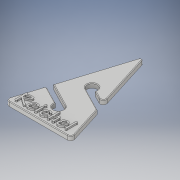
# Autodesk Inventor part: arrow_copied
Saved by Autodesk Inventor 2019 (Build 230136000, 136)
## iProperties
Created: 2019-04-04
Part Number: arrow_copied
Material: Generic
Document SubType Name: Modeling
Designer: jmc
Density: 1 g/cm^3
Appearance: Default
Author: jmc
Autodesk Inventor part; units mm, degrees
ref_plane "YZ Plane" through (0, 0, 0) normal (1, 0, 0) x (0, 1, 0)
ref_plane "XZ Plane" through (0, 0, 0) normal (0, 1, 0) x (-1, 0, 0)
ref_plane "XY Plane" through (0, 0, 0) normal (0, 0, 1) x (1, 0, 0)
sketch "Sketch1" plane through (0, 0, 0) normal (0, 1, 0) x (-1, 0, 0)
  line L0 (18.6404, 33.842) -> (-18.6393, 33.842)
  arc A0 (-0.9051, -31.4569) -> (1.0039, -31.4556) centre (0.0492, -31.158) ccw
  line L1 (-11.041, 0.8979) -> (-0.9051, -31.4569)
  line L2 (14.0042, 10.2488) -> (1.0039, -31.4556)
  arc A1 (20.5497, 31.2468) -> (18.6404, 33.842) centre (18.6404, 31.842) ccw
  arc A2 (-18.6393, 33.842) -> (-20.5478, 31.2441) centre (-18.6393, 31.842) ccw
  arc A3 (3.0063, 19.9469) -> (-1.4629, 18.1957) centre (-0.0005, 21.042) ccw
  arc A4 (-3.0072, 0.5972) -> (1.4619, 2.3483) centre (-0.0005, -0.498) ccw
  line L3 (14.0339, 14.281) -> (3.0063, 19.9469)
  line L4 (-1.4629, 18.1957) -> (14.0042, 10.2488)
  line L5 (20.5497, 31.2468) -> (15.4456, 14.8728)
  line L6 (14.0042, 10.2488) -> (1.0039, -31.4556)
  line L7 (1.4619, 2.3483) -> (-13.9812, 10.2829)
  line L8 (-3.0072, 0.5972) -> (-8.2185, 3.2747)
  line L9 (-20.5478, 31.2441) -> (-13.9812, 10.2829)
  line L10 (-11.041, 0.8979) -> (-0.9051, -31.4569)
  arc A5 (14.0339, 14.281) -> (15.4456, 14.8728) centre (14.4909, 15.1704) ccw
  arc A6 (-8.2185, 3.2747) -> (-11.041, 0.8979) centre (-9.1325, 1.4958) ccw
  point P0 (-0.0005, -4.3624)
  point P1 (-0.0005, -4.3624)
  point P2 (20.9995, 33.842)
  point P3 (21.3587, 33.842)
  point P4 (-21.3617, 33.842)
  point P5 (-0.0005, -4.3624)
  point P6 (-0.0005, 33.842)
  point P7 (-0.0005, -4.3624)
  point P8 (15.0916, 13.7375)
  point P9 (-12.47, 5.4591)
  dimension "d3" = 1
  dimension "d26" = 2
  dimension "d27" = 6.4
  dimension "d28" = 12.8
  dimension "d30" = 6.4
  dimension "d31" = 21.54
  dimension "d33" = 3.6
  dimension "d35" = 3.6
  dimension "d38" = 1
  dimension "d39" = 2
  constraints: 22 end point, 18 tangent, 14 point on circle, 9 point on line, 7 centre point, 3 coincident, 3 parallel, 1 equal radius, 1 horizontal
  measures "d3" radius of A0
  measures "d26" radius of A1
  measures "d27" diameter of A3
  measures "d28" distance from line of A3.centre L0
  measures "d30" diameter of A4
  measures "d31" distance of A4.centre A3.centre
  measures "d33" distance between parallel lines of L3 L4
  measures "d35" distance between parallel lines of L7 L8
  measures "d38" radius of A5
  measures "d39" radius of A6
extrude "Extrusion1" add sketch "Sketch1" along normal blind 2.8
sketch "Sketch2" plane through (0, 2.8, 0) normal (0, 1, 0) x (1, 0, 0)
  line L0 (-17.863, -24.2841) -> (16.586, -24.2841) construction
  line L1 (16.586, -24.2841) -> (16.586, -32.2942) construction
  line L2 (16.586, -32.2942) -> (-17.863, -32.2942) construction
  line L3 (-17.863, -32.2942) -> (-17.863, -24.2841) construction
  spline S0 degree 2 poles (-17.1698, -31.489) (-17.1698, -31.7411) (-16.9037, -32.1122) (-16.6096, -32.1192) knots 0 0 0 1 2 2 2
  spline S1 degree 2 poles (-16.6096, -32.1192) (-16.2946, -32.1262) (-15.8114, -31.8671) (-15.7974, -31.524) knots 0 0 0 1 2 2 2
  spline S2 degree 2 poles (-15.7974, -31.524) (-15.7974, -31.419) (-15.8744, -31.2159) (-15.9025, -31.1599) knots 0 0 0 1 2 2 2
  line L4 (-15.9025, -31.1599) -> (-15.9025, -28.8563)
  line L5 (-15.9025, -28.8563) -> (-11.7504, -31.8811)
  spline S3 degree 2 poles (-11.7504, -31.8811) (-11.6664, -32.0421) (-11.3653, -32.2032) (-11.1902, -32.2032) knots 0 0 0 1 2 2 2
  spline S4 degree 2 poles (-11.1902, -32.2032) (-10.9242, -32.2032) (-10.497, -31.8531) (-10.483, -31.51) knots 0 0 0 1 2 2 2
  spline S5 degree 2 poles (-10.483, -31.51) (-10.497, -31.2789) (-10.9452, -30.9359) (-11.2532, -31.0339) knots 0 0 0 1 2 2 2
  line L6 (-11.2532, -31.0339) -> (-15.0832, -28.2682)
  spline S6 degree 2 poles (-15.0832, -28.2682) (-13.2768, -27.9461) (-11.3653, -26.5947) (-11.3583, -25.6845) knots 0 0 0 1 2 2 2
  spline S7 degree 2 poles (-11.3583, -25.6845) (-11.3723, -25.0963) (-12.2685, -24.4662) (-13.0037, -24.4592) knots 0 0 0 1 2 2 2
  spline S8 degree 2 poles (-13.0037, -24.4592) (-13.7109, -24.4592) (-15.1533, -24.7813) (-15.9025, -25.1173) knots 0 0 0 1 2 2 2
  line L7 (-15.9025, -25.1173) -> (-15.9025, -24.9983)
  spline S9 degree 2 poles (-15.9025, -24.9983) (-15.8184, -24.6972) (-16.1405, -24.3261) (-16.4206, -24.3191) knots 0 0 0 1 2 2 2
  spline S10 degree 2 poles (-16.4206, -24.3191) (-16.6937, -24.3191) (-17.0858, -24.6132) (-17.0998, -24.8723) knots 0 0 0 1 2 2 2
  spline S11 degree 2 poles (-17.0998, -24.8723) (-17.0928, -24.9633) (-17.0437, -25.1524) (-17.0157, -25.2154) knots 0 0 0 1 2 2 2
  line L8 (-17.0157, -25.2154) -> (-17.0157, -25.4674)
  spline S12 degree 2 poles (-17.0157, -25.4674) (-17.1698, -25.5165) (-17.3798, -25.8315) (-17.3798, -26.1256) knots 0 0 0 1 2 2 2
  spline S13 degree 2 poles (-17.3798, -26.1256) (-17.3728, -26.3567) (-17.2118, -26.5807) (-17.1208, -26.5737) knots 0 0 0 1 2 2 2
  spline S14 degree 2 poles (-17.1208, -26.5737) (-17.0858, -26.5807) (-17.0367, -26.5667) (-17.0157, -26.5527) knots 0 0 0 1 2 2 2
  line L9 (-17.0157, -26.5527) -> (-17.0157, -31.1109)
  spline S15 degree 2 poles (-17.0157, -31.1109) (-17.0648, -31.1879) (-17.1628, -31.398) (-17.1698, -31.489) knots 0 0 0 1 2 2 2
  spline S16 degree 2 poles (-15.9025, -26.0276) (-15.1463, -25.6775) (-13.8159, -25.3834) (-13.3118, -25.3904) knots 0 0 0 1 2 2 2
  spline S17 degree 2 poles (-13.3118, -25.3904) (-12.9547, -25.3904) (-12.5416, -25.6355) (-12.5416, -25.8525) knots 0 0 0 1 2 2 2
  spline S18 degree 2 poles (-12.5416, -25.8525) (-12.5486, -26.2796) (-13.4518, -26.9588) (-14.9712, -27.491) (-15.9025, -27.687) knots 0 0 0 1 2 3 3 3
  line L10 (-15.9025, -27.687) -> (-15.9025, -26.0276)
  spline S19 degree 2 poles (-7.2132, -26.8118) (-8.0044, -26.8188) (-9.4048, -27.792) (-10.294, -29.4865) (-10.308, -30.5998) knots 0 0 0 1 2 3 3 3
  spline S20 degree 2 poles (-10.308, -30.5998) (-10.294, -31.496) (-9.3067, -32.2592) (-8.5365, -32.2522) knots 0 0 0 1 2 2 2
  spline S21 degree 2 poles (-8.5365, -32.2522) (-7.8084, -32.2382) (-6.7021, -31.8181) (-5.9529, -31.2159) (-5.5748, -30.6698) (-5.5748, -30.5368) knots 0 0 0 1 2 3 4 4 4
  spline S22 degree 2 poles (-5.5748, -30.5368) (-5.5678, -30.3477) (-5.7848, -30.0256) (-6.1069, -30.0186) knots 0 0 0 1 2 2 2
  spline S23 degree 2 poles (-6.1069, -30.0186) (-6.401, -30.0256) (-6.7161, -30.3267) (-6.6951, -30.5368) knots 0 0 0 1 2 2 2
  spline S24 degree 2 poles (-6.6951, -30.5368) (-6.8071, -30.7048) (-7.2972, -31.0689) (-7.9974, -31.321) (-8.4105, -31.328) knots 0 0 0 1 2 3 3 3
  spline S25 degree 2 poles (-8.4105, -31.328) (-8.7956, -31.335) (-9.2227, -30.9429) (-9.2227, -30.5017) knots 0 0 0 1 2 2 2
  spline S26 degree 2 poles (-9.2227, -30.5017) (-9.2227, -30.3267) (-9.1877, -30.0046) (-9.1387, -29.8646) knots 0 0 0 1 2 2 2
  line L11 (-9.1387, -29.8646) -> (-8.5996, -29.7666)
  spline S27 degree 2 poles (-8.5996, -29.7666) (-7.5773, -29.5915) (-6.331, -29.2204) (-5.7008, -28.8493) (-5.4837, -28.4712) (-5.4908, -28.2682) knots 0 0 0 1 2 3 4 4 4
  spline S28 degree 2 poles (-5.4908, -28.2682) (-5.4837, -28.0231) (-5.7988, -27.3509) (-6.555, -26.8258) (-7.2132, -26.8118) knots 0 0 0 1 2 3 3 3
  spline S29 degree 2 poles (-7.2622, -27.715) (-6.8771, -27.729) (-6.534, -28.0931) (-6.541, -28.3172) knots 0 0 0 1 2 2 2
  spline S30 degree 2 poles (-6.541, -28.3172) (-6.527, -28.4012) (-6.8631, -28.5902) (-7.8924, -28.8423) (-8.9286, -29.0244) knots 0 0 0 1 2 3 3 3
  spline S31 degree 2 poles (-8.9286, -29.0244) (-8.6556, -28.4502) (-7.7733, -27.729) (-7.2622, -27.715) knots 0 0 0 1 2 2 2
  spline S32 degree 2 poles (-3.1942, -27.4349) (-3.2012, -27.2389) (-3.5583, -26.8958) (-3.7753, -26.8818) knots 0 0 0 1 2 2 2
  spline S33 degree 2 poles (-3.7753, -26.8818) (-4.1254, -26.8888) (-4.4475, -27.0849) (-4.5245, -27.3999) (-4.5175, -27.568) knots 0 0 0 1 2 3 3 3
  spline S34 degree 2 poles (-4.5175, -27.568) (-4.5175, -27.652) (-4.4685, -27.82) (-4.4125, -27.8761) knots 0 0 0 1 2 2 2
  line L12 (-4.4125, -27.8761) -> (-4.4125, -31.1599)
  spline S35 degree 2 poles (-4.4125, -31.1599) (-4.4545, -31.2019) (-4.5525, -31.405) (-4.5525, -31.566) knots 0 0 0 1 2 2 2
  spline S36 degree 2 poles (-4.5525, -31.566) (-4.5525, -31.8251) (-4.2584, -32.1192) (-4.0204, -32.1192) knots 0 0 0 1 2 2 2
  spline S37 degree 2 poles (-4.0204, -32.1192) (-3.8313, -32.1192) (-3.4392, -31.9931) (-3.1661, -31.7411) (-3.1591, -31.538) knots 0 0 0 1 2 3 3 3
  spline S38 degree 2 poles (-3.1591, -31.538) (-3.1661, -31.433) (-3.2642, -31.2439) (-3.3132, -31.2089) knots 0 0 0 1 2 2 2
  line L13 (-3.3132, -31.2089) -> (-3.3132, -27.827)
  spline S39 degree 2 poles (-3.3132, -27.827) (-3.2922, -27.778) (-3.2012, -27.589) (-3.1942, -27.4349) knots 0 0 0 1 2 2 2
  spline S40 degree 2 poles (-3.7053, -24.6272) (-4.0414, -24.6412) (-4.4125, -25.2434) (-4.4125, -25.7055) knots 0 0 0 1 2 2 2
  spline S41 degree 2 poles (-4.4125, -25.7055) (-4.4125, -25.9576) (-4.1604, -26.2656) (-3.8803, -26.2726) knots 0 0 0 1 2 2 2
  spline S42 degree 2 poles (-3.8803, -26.2726) (-3.5933, -26.2656) (-3.1802, -25.6985) (-3.1732, -25.1734) knots 0 0 0 1 2 2 2
  spline S43 degree 2 poles (-3.1732, -25.1734) (-3.1732, -24.9143) (-3.4462, -24.6272) (-3.7053, -24.6272) knots 0 0 0 1 2 2 2
  spline S44 degree 2 poles (0.7829, -26.8118) (0.4608, -26.8188) (-0.2324, -27.0779) (-0.8275, -27.463) (-0.9956, -27.659) knots 0 0 0 1 2 3 3 3
  spline S45 degree 2 poles (-0.9956, -27.659) (-1.3527, -28.0091) (-1.8988, -28.7513) (-2.2069, -29.7035) (-2.2139, -30.3757) knots 0 0 0 1 2 3 3 3
  spline S46 degree 2 poles (-2.2139, -30.3757) (-2.2069, -31.2229) (-1.1986, -32.2732) (-0.3164, -32.2872) knots 0 0 0 1 2 2 2
  spline S47 degree 2 poles (-0.3164, -32.2872) (0.2297, -32.2872) (1.098, -31.9861) (1.4691, -31.6851) knots 0 0 0 1 2 2 2
  spline S48 degree 2 poles (1.4691, -31.6851) (1.8121, -31.433) (2.2673, -30.8588) (2.4983, -30.3967) (2.4983, -30.3267) knots 0 0 0 1 2 3 3 3
  spline S49 degree 2 poles (2.4983, -30.3267) (2.5053, -30.1797) (2.2533, -29.8436) (1.9242, -29.8296) knots 0 0 0 1 2 2 2
  spline S50 degree 2 poles (1.9242, -29.8296) (1.6441, -29.8366) (1.441, -30.1447) (1.399, -30.3827) knots 0 0 0 1 2 2 2
  spline S51 degree 2 poles (1.399, -30.3827) (1.28, -30.6068) (0.9019, -30.9779) (0.7059, -31.0969) knots 0 0 0 1 2 2 2
  spline S52 degree 2 poles (0.7059, -31.0969) (0.5238, -31.2019) (0.1527, -31.342) (-0.0503, -31.342) knots 0 0 0 1 2 2 2
  spline S53 degree 2 poles (-0.0503, -31.342) (-0.5895, -31.335) (-1.1286, -30.7398) (-1.1286, -30.1937) knots 0 0 0 1 2 2 2
  spline S54 degree 2 poles (-1.1286, -30.1937) (-1.1146, -29.5915) (-0.6175, -28.6253) (-0.3024, -28.3172) knots 0 0 0 1 2 2 2
  spline S55 degree 2 poles (-0.3024, -28.3172) (-0.0433, -28.0371) (0.5028, -27.729) (0.8109, -27.729) knots 0 0 0 1 2 2 2
  spline S56 degree 2 poles (0.8109, -27.729) (1.105, -27.736) (1.322, -27.9111) (1.364, -28.0231) knots 0 0 0 1 2 2 2
  spline S57 degree 2 poles (1.364, -28.0231) (1.406, -28.1281) (1.5531, -28.3032) (1.7421, -28.3102) knots 0 0 0 1 2 2 2
  spline S58 degree 2 poles (1.7421, -28.3102) (2.0992, -28.3032) (2.4283, -27.9881) (2.4283, -27.729) knots 0 0 0 1 2 2 2
  spline S59 degree 2 poles (2.4283, -27.729) (2.4143, -27.3439) (1.4831, -26.8258) (0.7829, -26.8118) knots 0 0 0 1 2 2 2
  spline S60 degree 2 poles (6.6994, -31.328) (6.6294, -31.405) (6.5804, -31.615) (6.5804, -31.7201) knots 0 0 0 1 2 2 2
  spline S61 degree 2 poles (6.5804, -31.7201) (6.5874, -31.9021) (6.9165, -32.1192) (7.1965, -32.1192) knots 0 0 0 1 2 2 2
  spline S62 degree 2 poles (7.1965, -32.1192) (7.4556, -32.1122) (7.8827, -31.8111) (7.8897, -31.601) knots 0 0 0 1 2 2 2
  spline S63 degree 2 poles (7.8897, -31.601) (7.8897, -31.524) (7.8127, -31.391) (7.7987, -31.342) knots 0 0 0 1 2 2 2
  line L14 (7.7987, -31.342) -> (7.7987, -28.0791)
  spline S64 degree 2 poles (7.7987, -28.0791) (7.8057, -27.484) (7.4346, -26.9098) (6.9725, -26.9098) knots 0 0 0 1 2 2 2
  spline S65 degree 2 poles (6.9725, -26.9098) (6.4894, -26.9098) (5.3341, -27.449) (4.7529, -27.9601) knots 0 0 0 1 2 2 2
  line L15 (4.7529, -27.9601) -> (4.7319, -27.9601)
  line L16 (4.7319, -27.9601) -> (4.7319, -25.1734)
  spline S66 degree 2 poles (4.7319, -25.1734) (4.7669, -25.0893) (4.8369, -24.9073) (4.8369, -24.8163) knots 0 0 0 1 2 2 2
  spline S67 degree 2 poles (4.8369, -24.8163) (4.8299, -24.6692) (4.6339, -24.4242) (4.3678, -24.2841) (4.2698, -24.2841) knots 0 0 0 1 2 3 3 3
  spline S68 degree 2 poles (4.2698, -24.2841) (3.9477, -24.2841) (3.5346, -24.5922) (3.5276, -24.8863) knots 0 0 0 1 2 2 2
  spline S69 degree 2 poles (3.5276, -24.8863) (3.5346, -24.9703) (3.6186, -25.1524) (3.6326, -25.2294) knots 0 0 0 1 2 2 2
  line L17 (3.6326, -25.2294) -> (3.6326, -31.349)
  spline S70 degree 2 poles (3.6326, -31.349) (3.5906, -31.405) (3.5486, -31.601) (3.5486, -31.7411) knots 0 0 0 1 2 2 2
  spline S71 degree 2 poles (3.5486, -31.7411) (3.5486, -31.9301) (3.7727, -32.1192) (4.0317, -32.1192) knots 0 0 0 1 2 2 2
  spline S72 degree 2 poles (4.0317, -32.1192) (4.3328, -32.1192) (4.8089, -31.8601) (4.8229, -31.636) knots 0 0 0 1 2 2 2
  spline S73 degree 2 poles (4.8229, -31.636) (4.8229, -31.531) (4.7739, -31.363) (4.7319, -31.307) knots 0 0 0 1 2 2 2
  line L18 (4.7319, -31.307) -> (4.7319, -29.1294)
  spline S74 degree 2 poles (4.7319, -29.1294) (5.236, -28.5132) (6.1743, -28.0511) (6.4403, -28.0651) knots 0 0 0 1 2 2 2
  spline S75 degree 2 poles (6.4403, -28.0651) (6.5874, -28.0581) (6.6994, -28.2822) (6.6994, -28.5832) knots 0 0 0 1 2 2 2
  line L19 (6.6994, -28.5832) -> (6.6994, -31.328)
  spline S76 degree 2 poles (11.9648, -26.8118) (11.1736, -26.8188) (9.7732, -27.792) (8.884, -29.4865) (8.87, -30.5998) knots 0 0 0 1 2 3 3 3
  spline S77 degree 2 poles (8.87, -30.5998) (8.884, -31.496) (9.8712, -32.2592) (10.6414, -32.2522) knots 0 0 0 1 2 2 2
  spline S78 degree 2 poles (10.6414, -32.2522) (11.3696, -32.2382) (12.4759, -31.8181) (13.2251, -31.2159) (13.6032, -30.6698) (13.6032, -30.5368) knots 0 0 0 1 2 3 4 4 4
  spline S79 degree 2 poles (13.6032, -30.5368) (13.6102, -30.3477) (13.3931, -30.0256) (13.0711, -30.0186) knots 0 0 0 1 2 2 2
  spline S80 degree 2 poles (13.0711, -30.0186) (12.777, -30.0256) (12.4619, -30.3267) (12.4829, -30.5368) knots 0 0 0 1 2 2 2
  spline S81 degree 2 poles (12.4829, -30.5368) (12.3709, -30.7048) (11.8808, -31.0689) (11.1806, -31.321) (10.7675, -31.328) knots 0 0 0 1 2 3 3 3
  spline S82 degree 2 poles (10.7675, -31.328) (10.3824, -31.335) (9.9553, -30.9429) (9.9553, -30.5017) knots 0 0 0 1 2 2 2
  spline S83 degree 2 poles (9.9553, -30.5017) (9.9553, -30.3267) (9.9903, -30.0046) (10.0393, -29.8646) knots 0 0 0 1 2 2 2
  line L20 (10.0393, -29.8646) -> (10.5784, -29.7666)
  spline S84 degree 2 poles (10.5784, -29.7666) (11.6007, -29.5915) (12.847, -29.2204) (13.4772, -28.8493) (13.6942, -28.4712) (13.6872, -28.2682) knots 0 0 0 1 2 3 4 4 4
  spline S85 degree 2 poles (13.6872, -28.2682) (13.6942, -28.0231) (13.3791, -27.3509) (12.6229, -26.8258) (11.9648, -26.8118) knots 0 0 0 1 2 3 3 3
  spline S86 degree 2 poles (11.9158, -27.715) (12.3009, -27.729) (12.644, -28.0931) (12.6369, -28.3172) knots 0 0 0 1 2 2 2
  spline S87 degree 2 poles (12.6369, -28.3172) (12.651, -28.4012) (12.3149, -28.5902) (11.2856, -28.8423) (10.2493, -29.0244) knots 0 0 0 1 2 3 3 3
  spline S88 degree 2 poles (10.2493, -29.0244) (10.5224, -28.4502) (11.4046, -27.729) (11.9158, -27.715) knots 0 0 0 1 2 2 2
  spline S89 degree 2 poles (14.7655, -31.2299) (14.7235, -31.314) (14.6605, -31.461) (14.6605, -31.538) knots 0 0 0 1 2 2 2
  spline S90 degree 2 poles (14.6605, -31.538) (14.6675, -31.8251) (15.0596, -32.1192) (15.3467, -32.1192) knots 0 0 0 1 2 2 2
  spline S91 degree 2 poles (15.3467, -32.1192) (15.6617, -32.1052) (16.0468, -31.7831) (16.0538, -31.622) knots 0 0 0 1 2 2 2
  spline S92 degree 2 poles (16.0538, -31.622) (16.0538, -31.524) (15.9628, -31.349) (15.8648, -31.2649) knots 0 0 0 1 2 2 2
  line L21 (15.8648, -31.2649) -> (15.8648, -25.3834)
  spline S93 degree 2 poles (15.8648, -25.3834) (15.9418, -25.2784) (16.0398, -25.0193) (16.0398, -24.8583) knots 0 0 0 1 2 2 2
  spline S94 degree 2 poles (16.0398, -24.8583) (16.0328, -24.5922) (15.6197, -24.3051) (15.3677, -24.3051) knots 0 0 0 1 2 2 2
  spline S95 degree 2 poles (15.3677, -24.3051) (14.9405, -24.2981) (14.6395, -24.5712) (14.6465, -24.9423) knots 0 0 0 1 2 2 2
  spline S96 degree 2 poles (14.6465, -24.9423) (14.6535, -25.0543) (14.7305, -25.2644) (14.7655, -25.3484) knots 0 0 0 1 2 2 2
  line L22 (14.7655, -25.3484) -> (14.7655, -31.2299)
  point P0 (0, 0)
  constraints: 2 other
extrude "Extrusion2" add sketch "Sketch2" along normal blind 1
fillet "Fillet1" radius 0.4 16 edges at (-0.0499, 2.8, -32.158) (5.9731, 2.8, -15.2795) (10.4208, 2.8, 3.0256) (5.6129, 2.8, 1.936) (-7.504, 2.8, -10.6034) (6.2596, 2.8, 6.3156) (-1.167, 2.8, -3.4774) (20.2511, 2.8, 33.0261) (-0.0005, 2.8, 33.842) (-20.2513, 2.8, 33.0273) (-17.9976, 2.8, 23.0598) (-14.8775, 2.8, 14.2482) (-8.5201, 2.8, 17.1139) (17.2645, 2.8, 20.7635) (-6.2706, 2.8, 14.2223) (1.1679, 2.8, 24.0215)
equation "\"d35\" = d33"
body "Solid1"
